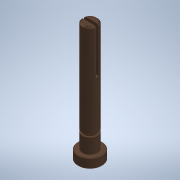
# Autodesk Inventor part: Wheel Handle
Saved by Autodesk Inventor 2021.1 (Build 251245010, 245A)
## iProperties
Created: 2025-09-16
Material: Bronze, Soft Tin
Document SubType Name: Modeling
Designer: SD
Density: 8.874 g/cm^3
Appearance: Bronze - Satin
Mass: 4.86247 g
Surface Area: 4.74167 cm^2
Volume: 0.547946 cm^3
Project: Automatic Tea Steeping mechanism
Part Number: Wheel Handle
Length: 37.000 mm
BOM-Mass: 0.00486
BOM-Area: 0.000
Diameter: 5.000 mm
Author: SD
Title: Wheel Handle
Autodesk Inventor part; units mm, degrees
ref_plane "YZ Plane" through (0, 0, 0) normal (1, 0, 0) x (0, 1, 0)
ref_plane "XZ Plane" through (0, 0, 0) normal (0, 1, 0) x (-1, 0, 0)
ref_plane "XY Plane" through (0, 0, 0) normal (0, 0, 1) x (1, 0, 0)
sketch "Sketch4" plane through (0, 0, 0) normal (0, 1, 0) x (-1, 0, 0)
  circle A0 centre (0, 0) radius 2.5
  constraints: 1 centre point, 1 coincident, 1 other
extrude "Extrusion2" add sketch "Sketch4" along normal mid plane 37
chamfer "Chamfer1" distance 0.5 angle 45 1 edges at (2.5, 18.5, 0)
sketch "Sketch14" plane through (0, -18.5, 0) normal (0, -1, 0) x (1, 0, 0)
  circle A0 centre (0, 0) radius 4
  dimension "d101" = 8
  constraints: 1 centre point, 1 coincident
  measures "d101" diameter of A0
extrude "Extrusion10" add sketch "Sketch14" along normal blind 3
sketch "Sketch15" plane through (0, 0, 0) normal (0, 0, 1) x (1, 0, 0)
  line L0 (-2.5, -18.5) -> (-2.5, 18) projected
  line L1 (-2.5, -12.7) -> (-2, -12.7)
  line L2 (-2, -12.7) -> (-2, -13.5)
  line L3 (-2, -13.5) -> (-2.5, -13.5)
  line L4 (-2.5, -13.5) -> (-2.5, -12.7)
  line L5 (0, -22.5133) -> (0, 22.052) construction
  line L6 (-4, -18.5) -> (4, -18.5) projected
  point P0 (0, 0)
  dimension "d104" = 2
  dimension "d105" = 0.8
  dimension "d106" = 5
  constraints: 10 end point, 2 parallel, 2 point on line, 1 horizontal, 1 perpendicular, 1 vertical
  measures "d104" distance between parallel lines of L2 L5
  measures "d105" distance between parallel lines of L3 L1
  measures "d106" distance between parallel lines of L6 L3
revolve "Revolution1" cut sketch "Sketch15" angle 360 about axis through (0, -22.5133, 0) along (0, 1, 0)
chamfer "Chamfer2" distance 0.1 angle 45 2 edges at (-4, -18.5, 0) (-4, -21.5, 0)
sketch "Sketch16" plane through (0, 0, 0) normal (1, 0, 0) x (0, 1, 0)
  line L0 (28.5, 0.5) -> (3.5, 0.5)
  line L1 (3.5, 0.5) -> (3.5, -0.5)
  line L2 (3.5, -0.5) -> (28.5, -0.5)
  line L3 (28.5, -0.5) -> (28.5, 0.5)
  line L4 (28.5, 0.5) -> (3.5, -0.5) construction
  line L5 (3.5, 0.5) -> (28.5, -0.5) construction
  line L6 (18.5, 2) -> (18.5, -2) projected
  point P0 (0, 0)
  point P1 (16, 0)
  dimension "d111" = 15
  dimension "d112" = 1
  dimension "d115" = 10
  constraints: 12 end point, 2 midpoint, 2 parallel, 1 horizontal, 1 horizontal alignment, 1 perpendicular
  measures "d111" distance between parallel lines of L1 L6
  measures "d112" distance between parallel lines of L0 L2
  measures "d115" distance between parallel lines of L3 L6
extrude "Extrusion11" cut sketch "Sketch16" against normal mid plane 7.75
body "Solid2"
